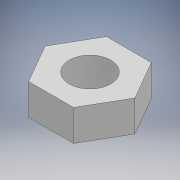
# Autodesk Inventor part: HexNut M4
Saved by Autodesk Inventor 2018.3 (Build 223284000, 284)
## iProperties
Created: 2020-03-30
Part Number: HexNut M4
Material: Generic
Document SubType Name: Modeling
Designer: Ivan
Density: 1 g/cm^3
Appearance: Default
Author: Ivan
Autodesk Inventor part; units mm, degrees
ref_plane "YZ Plane" through (0, 0, 0) normal (1, 0, 0) x (0, 1, 0)
ref_plane "XZ Plane" through (0, 0, 0) normal (0, 1, 0) x (-1, 0, 0)
ref_plane "XY Plane" through (0, 0, 0) normal (0, 0, 1) x (1, 0, 0)
sketch "Sketch1" plane through (0, 0, 0) normal (0, 0, 1) x (1, 0, 0)
  line L0 (2.1651, -3.75) -> (-2.1651, -3.75)
  line L1 (-2.1651, -3.75) -> (-4.3301, 0)
  line L2 (-4.3301, 0) -> (-2.1651, 3.75)
  line L3 (-2.1651, 3.75) -> (2.1651, 3.75)
  line L4 (2.1651, 3.75) -> (4.3301, 0)
  line L5 (4.3301, 0) -> (2.1651, -3.75)
  circle A0 centre (0, 0) radius 2
  line L6 (-6.0622, 0) -> (6.0622, 0) construction
  dimension "d0" = 7.5
  dimension "d1" = 4
  constraints: 12 end point, 2 coincident, 1 centre point, 1 parallel, 13 other
  measures "d0" distance between parallel lines of L0 L3
  measures "d1" diameter of A0
extrude "Extrusion1" add sketch "Sketch1" along normal blind 3
body "Solid1"
